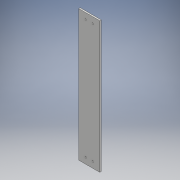
# Autodesk Inventor part: platen_286mm
Saved by Autodesk Inventor 2018 (Build 220112000, 112)
## iProperties
Created: 2018-10-27
Part Number: platen_286mm
Material: Generic
Document SubType Name: Modeling
Designer: Fredy Espana C
Density: 1 g/cm^3
Appearance: Default
Author: Fredy Espana C
Autodesk Inventor part; units mm, degrees
ref_plane "YZ Plane" through (0, 0, 0) normal (1, 0, 0) x (0, 1, 0)
ref_plane "XZ Plane" through (0, 0, 0) normal (0, 1, 0) x (-1, 0, 0)
ref_plane "XY Plane" through (0, 0, 0) normal (0, 0, 1) x (1, 0, 0)
sketch "Sketch1" plane through (0, 0, 0) normal (0, 0, 1) x (1, 0, 0)
  line L0 (0, 0) -> (44.45, 0)
  line L1 (44.45, 0) -> (44.45, 3.175)
  line L2 (44.45, 3.175) -> (0, 3.175)
  line L3 (0, 3.175) -> (0, 0)
  dimension "d0" = 44.45
  dimension "d1" = 3.175
  constraints: 8 end point, 2 parallel, 1 horizontal, 1 perpendicular
  measures "d0" distance of L0.start L0.end
  measures "d1" distance of L2.end L0.start
extrude "Extrusion1" add sketch "Sketch1" along normal blind 276
sketch "Sketch2" plane through (0, 0, 0) normal (0, -1, 0) x (1, 0, 0)
  line L0 (0, 0) -> (44.45, 0) projected
  line L1 (44.45, 0) -> (44.45, 276) projected
  line L2 (0, 276) -> (44.45, 276) projected
  line L3 (0, 0) -> (0, 276) projected
  point P0 (14.81, 263.3)
  point P1 (29.62, 263.3)
  point P2 (14.81, 12.7)
  point P3 (29.62, 12.7)
  dimension "d4" = 12.7
  dimension "d5" = 12.7
  dimension "d6" = 14.81
  dimension "d7" = 14.81
  constraints: 2 horizontal alignment, 2 vertical alignment
  measures "d4" distance from line of point (14.81, 263.3) L2
  measures "d5" distance from line of point (14.81, 12.7) L0
  measures "d6" distance of point (29.62, 12.7) point (14.81, 12.7)
  measures "d7" distance from line of L3 point (14.81, 12.7)
hole "Hole1" at (14.81, 0, 263.3) at (29.62, 0, 263.3) at (14.81, 0, 12.7) at (29.62, 0, 12.7) direction (0, 1, 0) diameter 3.175 depth 8 tip angle 118
body "Solid1"
